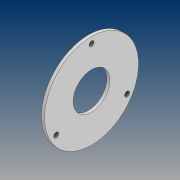
# Autodesk Inventor part: AsfaleiaDIpteroy
Saved by Autodesk Inventor 2021 (Build 250183000, 183)
## iProperties
Created: 2021-01-09
Part Number: AsfaleiaDIpteroy
Material: Generic
Document SubType Name: Modeling
Designer: Διογενης Τσιχλακης
Density: 1 g/cm^3
Appearance: Default
Author: Διογενης Τσιχλακης
Autodesk Inventor part; units mm, degrees
ref_plane "YZ Plane" through (0, 0, 0) normal (1, 0, 0) x (0, 1, 0)
ref_plane "XZ Plane" through (0, 0, 0) normal (0, 1, 0) x (-1, 0, 0)
ref_plane "XY Plane" through (0, 0, 0) normal (0, 0, 1) x (1, 0, 0)
sketch "Sketch1" plane through (0, 0, 0) normal (1, 0, 0) x (0, 1, 0)
  circle A0 centre (0, 0) radius 30
  circle A1 centre (0, 0) radius 76.45
  dimension "d11" = 152.9
  dimension "d12" = 60
  constraints: 2 centre point
  measures "d11" diameter of A1
  measures "d12" diameter of A0
extrude "Extrusion1" add sketch "Sketch1" along normal blind 5
sketch "Sketch3" plane through (5, 0, 0) normal (1, 0, 0) x (0, 0, -1)
  circle A0 centre (0, 0) radius 66.5
  circle A1 centre (0, 66.5) radius 4
  circle A2 centre (-57.5907, -33.25) radius 4
  circle A3 centre (57.5907, -33.25) radius 4
  dimension "d23" = 133
  dimension "d24" = 8
  dimension "d45" = 360
  constraints: 3 centre point, 1 coincident, 1 vertical alignment, 9 other
  measures "d24" diameter of A1
extrude "Extrusion4" cut sketch "Sketch3" against normal through all contours A1 A0 | A0 A1 | A3 A0 | A0 A3 | A2 A0 | A0 A2
thread "Thread1" size "M8x1.25" class "6H" standard "ANSI Metric M Profile" full length
thread "Thread5" size "M8x1.25" class "6H" standard "ANSI Metric M Profile" full length
thread "Thread6" size "M8x1.25" class "6H" standard "ANSI Metric M Profile" full length
body "Solid1"
